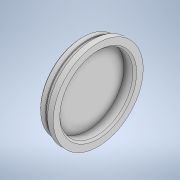
# Autodesk Inventor part: Крышка, тихая
Saved by Autodesk Inventor 2021 (Build 250183000, 183)
## iProperties
Created: 2023-03-17
Part Number: Крышка, тихая
Material: Типовые
Document SubType Name: Modeling
Designer: gdevc
Density: 1 g/cm^3
Appearance: По умолчанию
Author: gdevc
Autodesk Inventor part; units mm, degrees
ref_plane "YZ Plane" through (0, 0, 0) normal (1, 0, 0) x (0, 1, 0)
ref_plane "XZ Plane" through (0, 0, 0) normal (0, 1, 0) x (-1, 0, 0)
ref_plane "XY Plane" through (0, 0, 0) normal (0, 0, 1) x (1, 0, 0)
sketch "Эскиз1" plane through (0, 0, 0) normal (0, 0, 1) x (1, 0, 0)
  line L0 (0, 0) -> (0, 45)
  line L1 (0, 45) -> (6, 45)
  line L2 (6, 45) -> (6.5, 44.5)
  line L3 (6.5, 44.5) -> (11.5, 44.5)
  line L4 (11.5, 44.5) -> (11.5, 48)
  line L5 (11.5, 48) -> (17.5, 48)
  line L6 (17.5, 48) -> (17.5, 39)
  line L7 (17.5, 39) -> (6, 39)
  line L8 (6, 39) -> (6, 0)
  line L9 (6, 0) -> (0, 0)
  dimension "d0" = 6
  dimension "d1" = 90
  dimension "d2" = 6
  dimension "d3" = 9
  dimension "d4" = 6
  dimension "d5" = 5
  dimension "d6" = 0.5
  dimension "d7" = 45
  dimension "d8" = 6
  dimension "d18" = 17.5
  constraints: 20 end point, 7 perpendicular, 1 parallel, 1 vertical
  measures "d0" distance between parallel lines of L0 L8
  measures "d1" diameter of L1 L9
  measures "d2" distance between parallel lines of L7 L1
  measures "d3" distance between parallel lines of L7 L5
  measures "d4" distance of L0.end L1.end
  measures "d5" distance of L2.end L3.end
  measures "d6" distance between parallel lines of L3 L1
  measures "d7" angle of L1 L2
  measures "d8" distance of L4.end L5.end
  measures "d18" distance between parallel lines of L6 L0
revolve "Вращение1" add sketch "Эскиз1" angle 360 about axis through (6, 0, 0) along (-1, 0, 0)
chamfer "Фаска1" distance 2 angle 45 1 edges at (17.5, -39, 0)
fillet "Сопряжение1" radius 0.5 1 edges at (6.5, -44.5, 0)
fillet "Сопряжение2" radius 1.6 1 edges at (11.5, -44.5, 0)
chamfer "Фаска2" distance 1 angle 45 1 edges at (0, -45, 0)
equation "\"d3\" = 1.5 * d2"
